Autodesk Fusion 360 part; units mm, degrees
(part 3 of 4)
  spline S780 degree 3 poles (162.707, 0) (162.5525, 0.1099) (162.343, 0.1683) (162.2434, 0.3296) knots 0 0 0 0 1 1 1 1
  spline S781 degree 3 poles (162.2434, 0.3296) (161.8581, 0.9535) (161.6678, 1.6847) (161.2818, 2.3082) knots 0 0 0 0 1 1 1 1
  spline S782 degree 3 poles (161.2818, 2.3082) (160.719, 3.2174) (160.1131, 4.1081) (159.4072, 4.9112) knots 0 0 0 0 1 1 1 1
  spline S783 degree 3 poles (159.4072, 4.9112) (158.7995, 5.6026) (158.0938, 6.2084) (157.3624, 6.7673) knots 0 0 0 0 1 1 1 1
  spline S784 degree 3 poles (157.3624, 6.7673) (156.5565, 7.3833) (155.641, 7.8427) (154.8102, 8.4245) knots 0 0 0 0 1 1 1 1
  spline S785 degree 3 poles (154.8102, 8.4245) (154.6015, 8.5707) (154.3988, 8.7382) (154.2513, 8.9459) knots 0 0 0 0 1 1 1 1
  spline S786 degree 3 poles (154.2513, 8.9459) (154.1313, 9.1149) (154.0733, 9.3238) (154.028, 9.526) knots 0 0 0 0 1 1 1 1
  spline S787 degree 3 poles (154.028, 9.526) (153.9612, 9.8241) (153.9281, 10.1306) (153.9173, 10.4359) knots 0 0 0 0 1 1 1 1
  spline S788 degree 3 poles (153.9173, 10.4359) (153.8511, 12.3143) (153.8373, 14.1943) (153.7972, 16.0734) knots 0 0 0 0 1 1 1 1
  spline S789 degree 3 poles (154.328, 36.0186) (154.1191, 36.017) (153.9103, 36.0154) (153.7014, 36.0138) knots 0 0 0 0 1 1 1 1
  spline S790 degree 3 poles (153.503, 90.7209) (153.3923, 90.7448) (153.2816, 90.7686) (153.1709, 90.7925) knots 0 0 0 0 1 1 1 1
  spline S791 degree 3 poles (153.0996, 107.2371) (153.1846, 106.7302) (153.3367, 106.2301) (153.3546, 105.7164) knots 0 0 0 0 1 1 1 1
  spline S792 degree 3 poles (153.3546, 105.7164) (153.416, 103.9626) (153.3139, 102.2065) (153.337, 100.4517) knots 0 0 0 0 1 1 1 1
  spline S793 degree 3 poles (153.337, 100.4517) (153.369, 98.0177) (153.5698, 95.5852) (153.5198, 93.1515) knots 0 0 0 0 1 1 1 1
  spline S794 degree 3 poles (153.5198, 93.1515) (153.5098, 92.6629) (153.2785, 92.2042) (153.1579, 91.7306) knots 0 0 0 0 1 1 1 1
  spline S795 degree 3 poles (153.0696, 113.8009) (153.1646, 113.374) (153.2945, 112.9533) (153.3547, 112.5201) knots 0 0 0 0 1 1 1 1
  spline S796 degree 3 poles (153.3547, 112.5201) (153.3831, 112.3158) (153.3687, 112.1048) (153.3337, 111.9015) knots 0 0 0 0 1 1 1 1
  spline S797 degree 3 poles (153.3337, 111.9015) (153.2775, 111.5746) (153.1664, 111.2595) (153.0827, 110.9385) knots 0 0 0 0 1 1 1 1
  spline S798 degree 3 poles (152.9654, 140.9767) (153.0459, 140.643) (153.1607, 140.3156) (153.2067, 139.9754) knots 0 0 0 0 1 1 1 1
  spline S799 degree 3 poles (153.2067, 139.9754) (153.2508, 139.6494) (153.2325, 139.3179) (153.2341, 138.9889) knots 0 0 0 0 1 1 1 1
  spline S800 degree 3 poles (153.2341, 138.9889) (153.2588, 133.9022) (153.2897, 128.8155) (153.2858, 123.7287) knots 0 0 0 0 1 1 1 1
  spline S801 degree 3 poles (153.2858, 123.7287) (153.2852, 123.0168) (153.2686, 122.3043) (153.2205, 121.5941) knots 0 0 0 0 1 1 1 1
  spline S802 degree 3 poles (153.2205, 121.5941) (153.1866, 121.0943) (153.0705, 120.6021) (153.04, 120.1021) knots 0 0 0 0 1 1 1 1
  spline S803 degree 3 poles (153.04, 120.1021) (153.0124, 119.6503) (153.0023, 119.1947) (153.0465, 118.7443) knots 0 0 0 0 1 1 1 1
  spline S804 degree 3 poles (153.0465, 118.7443) (153.1022, 118.1763) (153.2777, 117.6248) (153.3386, 117.0573) knots 0 0 0 0 1 1 1 1
  spline S805 degree 3 poles (153.3386, 117.0573) (153.3709, 116.7565) (153.3702, 116.4489) (153.3248, 116.1498) knots 0 0 0 0 1 1 1 1
  spline S806 degree 3 poles (153.3248, 116.1498) (153.2775, 115.8382) (153.1502, 115.544) (153.0629, 115.2411) knots 0 0 0 0 1 1 1 1
  spline S807 degree 3 poles (154.0634, 122.5487) (153.7954, 122.5914) (153.5274, 122.6342) (153.2594, 122.677) knots 0 0 0 0 1 1 1 1
  spline S808 degree 3 poles (152.9512, 147.0062) (153.0349, 146.6532) (153.1573, 146.3072) (153.2024, 145.9472) knots 0 0 0 0 1 1 1 1
  spline S809 degree 3 poles (153.2024, 145.9472) (153.2487, 145.5771) (153.223, 145.2015) (153.2237, 144.8285) knots 0 0 0 0 1 1 1 1
  spline S810 degree 3 poles (153.2237, 144.8285) (153.2242, 144.5201) (153.2505, 144.2085) (153.206, 143.9033) knots 0 0 0 0 1 1 1 1
  spline S811 degree 3 poles (153.206, 143.9033) (153.1619, 143.602) (153.042, 143.3168) (152.96, 143.0235) knots 0 0 0 0 1 1 1 1
  spline S812 degree 3 poles (152.9452, 150.8938) (153.0274, 150.6921) (153.1451, 150.5015) (153.192, 150.2887) knots 0 0 0 0 1 1 1 1
  spline S813 degree 3 poles (153.192, 150.2887) (153.2367, 150.086) (153.2152, 149.874) (153.2156, 149.6664) knots 0 0 0 0 1 1 1 1
  spline S814 degree 3 poles (153.2156, 149.6664) (153.2159, 149.5184) (153.2239, 149.368) (153.1941, 149.223) knots 0 0 0 0 1 1 1 1
  spline S815 degree 3 poles (153.1941, 149.223) (153.1344, 148.9333) (153.0305, 148.6545) (152.9488, 148.3703) knots 0 0 0 0 1 1 1 1
  spline S816 degree 3 poles (156.3329, 165.4136) (156.0015, 165.2513) (155.6952, 165.0222) (155.3388, 164.9267) knots 0 0 0 0 1 1 1 1
  spline S817 degree 3 poles (155.3388, 164.9267) (155.0427, 164.8474) (154.7258, 164.886) (154.4196, 164.9012) knots 0 0 0 0 1 1 1 1
  spline S818 degree 3 poles (154.4196, 164.9012) (154.1292, 164.9157) (153.843, 164.9775) (153.5547, 165.0156) knots 0 0 0 0 1 1 1 1
  spline S819 degree 3 poles (155.7861, 165.1661) (155.9235, 165.0932) (156.044, 164.9681) (156.1982, 164.9473) knots 0 0 0 0 1 1 1 1
  spline S820 degree 3 poles (156.1982, 164.9473) (156.6531, 164.8858) (157.1161, 164.9234) (157.5752, 164.9243) knots 0 0 0 0 1 1 1 1
  spline S821 degree 3 poles (157.5752, 164.9243) (157.8528, 164.9248) (158.1321, 164.9161) (158.4074, 164.9514) knots 0 0 0 0 1 1 1 1
  spline S822 degree 3 poles (158.4074, 164.9514) (158.8796, 165.012) (159.3437, 165.1247) (159.8118, 165.2113) knots 0 0 0 0 1 1 1 1
  spline S823 degree 3 poles (178.3424, 165.3678) (177.9374, 165.3072) (177.5356, 165.2189) (177.1274, 165.1861) knots 0 0 0 0 1 1 1 1
  spline S824 degree 3 poles (177.1274, 165.1861) (176.75, 165.1558) (176.3688, 165.1469) (175.9915, 165.1789) knots 0 0 0 0 1 1 1 1
  spline S825 degree 3 poles (175.9915, 165.1789) (175.5602, 165.2155) (175.1431, 165.3827) (174.7102, 165.391) knots 0 0 0 0 1 1 1 1
  spline S826 degree 3 poles (174.7102, 165.391) (172.3795, 165.4359) (170.0478, 165.2968) (167.717, 165.3382) knots 0 0 0 0 1 1 1 1
  spline S827 degree 3 poles (167.717, 165.3382) (167.2356, 165.3468) (166.767, 165.5072) (166.2867, 165.5408) knots 0 0 0 0 1 1 1 1
  spline S828 degree 3 poles (166.2867, 165.5408) (165.7509, 165.5783) (165.2126, 165.5544) (164.6756, 165.551) knots 0 0 0 0 1 1 1 1
  spline S829 degree 3 poles (164.6756, 165.551) (163.9812, 165.5467) (163.284, 165.5818) (162.5925, 165.5178) knots 0 0 0 0 1 1 1 1
  spline S830 degree 3 poles (162.5925, 165.5178) (162.3658, 165.4968) (162.1614, 165.3716) (161.9459, 165.2984) knots 0 0 0 0 1 1 1 1
  spline S831 degree 3 poles (179.1031, 165.3338) (178.8495, 165.3452) (178.5938, 165.3331) (178.3424, 165.3678) knots 0 0 0 0 1 1 1 1
  spline S832 degree 3 poles (178.3424, 165.3678) (177.8191, 165.44) (177.309, 165.5983) (176.7837, 165.6538) knots 0 0 0 0 1 1 1 1
  spline S833 degree 3 poles (176.7837, 165.6538) (176.47, 165.687) (176.1487, 165.6841) (175.8375, 165.6326) knots 0 0 0 0 1 1 1 1
  spline S834 degree 3 poles (175.8375, 165.6326) (175.6902, 165.6081) (175.5709, 165.498) (175.4375, 165.4307) knots 0 0 0 0 1 1 1 1
  spline S835 degree 3 poles (179.0957, 165.9568) (179.1114, 159.0174) (179.1975, 152.0777) (179.143, 145.1384) knots 0 0 0 0 1 1 1 1
  spline S836 degree 3 poles (179.143, 145.1384) (179.1379, 144.4898) (178.9671, 143.8524) (178.917, 143.2057) knots 0 0 0 0 1 1 1 1
  spline S837 degree 3 poles (178.917, 143.2057) (178.8989, 142.9714) (178.8909, 142.731) (178.9388, 142.5009) knots 0 0 0 0 1 1 1 1
  spline S838 degree 3 poles (178.9388, 142.5009) (179.046, 141.9849) (179.2688, 141.4978) (179.3792, 140.9825) knots 0 0 0 0 1 1 1 1
  spline S839 degree 3 poles (179.3792, 140.9825) (179.43, 140.7456) (179.4179, 140.499) (179.4196, 140.2568) knots 0 0 0 0 1 1 1 1
  spline S840 degree 3 poles (179.4196, 140.2568) (179.4248, 139.496) (179.4847, 138.7306) (179.3998, 137.9747) knots 0 0 0 0 1 1 1 1
  spline S841 degree 3 poles (179.3998, 137.9747) (179.3234, 137.2945) (179.055, 136.6483) (178.9383, 135.974) knots 0 0 0 0 1 1 1 1
  spline S842 degree 3 poles (178.9383, 135.974) (178.8948, 135.7226) (178.9209, 135.4639) (178.9211, 135.2088) knots 0 0 0 0 1 1 1 1
  spline S843 degree 3 poles (178.9211, 135.2088) (178.9271, 127.7745) (178.9353, 120.3402) (178.957, 112.9059) knots 0 0 0 0 1 1 1 1
  spline S844 degree 3 poles (178.957, 112.9059) (178.9581, 112.5277) (178.9443, 112.1473) (178.9892, 111.7717) knots 0 0 0 0 1 1 1 1
  spline S845 degree 3 poles (178.9892, 111.7717) (179.0311, 111.4216) (179.1404, 111.0828) (179.2161, 110.7384) knots 0 0 0 0 1 1 1 1
  spline S846 degree 3 poles (179.143, 145.1384) (179.2272, 144.7257) (179.3417, 144.3182) (179.3955, 143.9005) knots 0 0 0 0 1 1 1 1
  spline S847 degree 3 poles (179.3955, 143.9005) (179.4332, 143.6079) (179.4218, 143.3106) (179.4166, 143.0156) knots 0 0 0 0 1 1 1 1
  spline S848 degree 3 poles (179.4166, 143.0156) (179.4127, 142.797) (179.4165, 142.5747) (179.3684, 142.3615) knots 0 0 0 0 1 1 1 1
  spline S849 degree 3 poles (179.3684, 142.3615) (179.2573, 141.8686) (178.9997, 141.4091) (178.9411, 140.9074) knots 0 0 0 0 1 1 1 1
  spline S850 degree 3 poles (178.9411, 140.9074) (178.8484, 140.1134) (178.9181, 139.3087) (178.9183, 138.5094) knots 0 0 0 0 1 1 1 1
  spline S851 degree 3 poles (178.9183, 138.5094) (178.9184, 138.3273) (178.9065, 138.1423) (178.942, 137.9638) knots 0 0 0 0 1 1 1 1
  spline S852 degree 3 poles (178.942, 137.9638) (179.0571, 137.3857) (179.2568, 136.8265) (179.3685, 136.2478) knots 0 0 0 0 1 1 1 1
  spline S853 degree 3 poles (179.3685, 136.2478) (179.4172, 135.996) (179.4206, 135.7367) (179.4215, 135.4802) knots 0 0 0 0 1 1 1 1
  spline S854 degree 3 poles (179.4215, 135.4802) (179.4469, 128.2535) (179.4502, 121.0268) (179.4474, 113.8001) knots 0 0 0 0 1 1 1 1
  spline S855 degree 3 poles (179.4474, 113.8001) (179.4472, 113.1228) (179.4861, 112.4418) (179.4125, 111.7686) knots 0 0 0 0 1 1 1 1
  spline S856 degree 3 poles (179.4125, 111.7686) (179.3245, 110.9633) (179.0168, 110.1885) (178.9642, 109.3801) knots 0 0 0 0 1 1 1 1
  spline S857 degree 3 poles (178.9642, 109.3801) (178.863, 107.8263) (178.9502, 106.2659) (178.9529, 104.7089) knots 0 0 0 0 1 1 1 1
  spline S858 degree 3 poles (178.9529, 104.7089) (178.9535, 104.3678) (178.9307, 104.0242) (178.9743, 103.686) knots 0 0 0 0 1 1 1 1
  spline S859 degree 3 poles (178.9743, 103.686) (179.0287, 103.2634) (179.1552, 102.8532) (179.2457, 102.4368) knots 0 0 0 0 1 1 1 1
  spline S860 degree 3 poles (179.3943, 127.6548) (179.2509, 127.6546) (179.1075, 127.6543) (178.9641, 127.6541) knots 0 0 0 0 1 1 1 1
  spline S861 degree 3 poles (179.2172, 110.3815) (179.2954, 110.0078) (179.4356, 109.6417) (179.4517, 109.2602) knots 0 0 0 0 1 1 1 1
  spline S862 degree 3 poles (179.4517, 109.2602) (179.5211, 107.6185) (179.5224, 105.9731) (179.4728, 104.3306) knots 0 0 0 0 1 1 1 1
  spline S863 degree 3 poles (179.4728, 104.3306) (179.4536, 103.6951) (179.2605, 103.0724) (179.2457, 102.4368) knots 0 0 0 0 1 1 1 1
  spline S864 degree 3 poles (179.2457, 102.4368) (179.1941, 100.2162) (179.3217, 97.9939) (179.274, 95.7732) knots 0 0 0 0 1 1 1 1
  spline S865 degree 3 poles (179.274, 95.7732) (179.2685, 95.5153) (179.1174, 95.2786) (179.0865, 95.0225) knots 0 0 0 0 1 1 1 1
  spline S866 degree 3 poles (179.0865, 95.0225) (179.0451, 94.6809) (179.059, 94.3346) (179.0585, 93.9905) knots 0 0 0 0 1 1 1 1
  spline S867 degree 3 poles (179.0585, 93.9905) (179.0537, 90.882) (179.0579, 87.7735) (179.0705, 84.665) knots 0 0 0 0 1 1 1 1
  spline S868 degree 3 poles (179.0705, 84.665) (179.0755, 83.4488) (179.0424, 82.2309) (179.1112, 81.0166) knots 0 0 0 0 1 1 1 1
  spline S869 degree 3 poles (179.1112, 81.0166) (179.1447, 80.4248) (179.2882, 79.8443) (179.3767, 79.2582) knots 0 0 0 0 1 1 1 1
  spline S870 degree 3 poles (179.274, 95.7732) (179.3589, 95.4159) (179.5199, 95.0684) (179.5286, 94.7013) knots 0 0 0 0 1 1 1 1
  spline S871 degree 3 poles (179.5286, 94.7013) (179.624, 90.6448) (179.5785, 86.5862) (179.5855, 82.5286) knots 0 0 0 0 1 1 1 1
  spline S872 degree 3 poles (179.5855, 82.5286) (179.5867, 81.862) (179.5956, 81.1942) (179.5532, 80.5289) knots 0 0 0 0 1 1 1 1
  spline S873 degree 3 poles (179.5532, 80.5289) (179.5259, 80.1022) (179.3964, 79.6854) (179.3767, 79.2582) knots 0 0 0 0 1 1 1 1
  spline S874 degree 3 poles (179.3767, 79.2582) (179.3439, 78.5443) (179.4327, 77.8281) (179.3962, 77.1144) knots 0 0 0 0 1 1 1 1
  spline S875 degree 3 poles (179.3962, 77.1144) (179.3745, 76.6904) (179.2124, 76.2799) (179.2027, 75.8554) knots 0 0 0 0 1 1 1 1
  spline S876 degree 3 poles (179.2027, 75.8554) (179.1504, 73.5649) (179.1994, 71.2732) (179.2105, 68.9821) knots 0 0 0 0 1 1 1 1
  spline S877 degree 3 poles (179.2105, 68.9821) (179.2136, 68.3531) (179.1876, 67.7218) (179.2452, 67.0955) knots 0 0 0 0 1 1 1 1
  spline S878 degree 3 poles (179.2452, 67.0955) (179.2874, 66.6365) (179.4209, 66.1907) (179.5088, 65.7383) knots 0 0 0 0 1 1 1 1
  spline S879 degree 3 poles (179.437, 69.1097) (179.528, 68.7981) (179.6191, 68.4865) (179.7101, 68.1749) knots 0 0 0 0 1 1 1 1
  spline S880 degree 3 poles (179.5184, 64.722) (179.4564, 64.4417) (179.3646, 64.1664) (179.3325, 63.8811) knots 0 0 0 0 1 1 1 1
  spline S881 degree 3 poles (179.3325, 63.8811) (179.2722, 63.3457) (179.1737, 62.8017) (179.242, 62.2673) knots 0 0 0 0 1 1 1 1
  spline S882 degree 3 poles (179.242, 62.2673) (179.3331, 61.5535) (179.6394, 60.8835) (179.8049, 60.1831) knots 0 0 0 0 1 1 1 1
  spline S883 degree 3 poles (179.8049, 60.1831) (179.833, 60.0641) (179.8201, 59.9389) (179.8211, 59.8165) knots 0 0 0 0 1 1 1 1
  spline S884 degree 3 poles (179.8211, 59.8165) (179.844, 57.0288) (179.867, 54.241) (179.8765, 51.4531) knots 0 0 0 0 1 1 1 1
  spline S885 degree 3 poles (179.8765, 51.4531) (179.8774, 51.2037) (179.8863, 50.9523) (179.8523, 50.7052) knots 0 0 0 0 1 1 1 1
  spline S886 degree 3 poles (179.8523, 50.7052) (179.81, 50.397) (179.6854, 50.1033) (179.6485, 49.7944) knots 0 0 0 0 1 1 1 1
  spline S887 degree 3 poles (179.6485, 49.7944) (179.6191, 49.5484) (179.6525, 49.2989) (179.6548, 49.0512) knots 0 0 0 0 1 1 1 1
  spline S888 degree 3 poles (179.6548, 49.0512) (179.657, 48.8038) (179.6345, 48.555) (179.6618, 48.3091) knots 0 0 0 0 1 1 1 1
  spline S889 degree 3 poles (179.6618, 48.3091) (179.7288, 47.7071) (179.9183, 47.1183) (179.9372, 46.5128) knots 0 0 0 0 1 1 1 1
  spline S890 degree 3 poles (179.9372, 46.5128) (180.0188, 43.89) (180.0047, 41.2644) (179.9627, 38.6406) knots 0 0 0 0 1 1 1 1
  spline S891 degree 3 poles (179.9627, 38.6406) (179.9546, 38.1306) (179.7698, 37.6304) (179.7869, 37.1206) knots 0 0 0 0 1 1 1 1
  spline S892 degree 3 poles (179.7869, 37.1206) (179.7941, 36.9044) (179.9871, 36.7317) (180.0336, 36.5204) knots 0 0 0 0 1 1 1 1
  spline S893 degree 3 poles (180.0336, 36.5204) (180.083, 36.2966) (180.0682, 36.063) (180.0704, 35.8337) knots 0 0 0 0 1 1 1 1
  spline S894 degree 3 poles (180.0704, 35.8337) (180.0975, 32.9366) (180.1603, 30.0391) (180.1215, 27.1421) knots 0 0 0 0 1 1 1 1
  spline S895 degree 3 poles (180.1215, 27.1421) (180.1103, 26.304) (179.961, 25.4728) (179.9205, 24.6356) knots 0 0 0 0 1 1 1 1
  spline S896 degree 3 poles (179.9205, 24.6356) (179.8989, 24.1883) (179.9658, 23.7391) (179.9354, 23.2923) knots 0 0 0 0 1 1 1 1
  spline S897 degree 3 poles (179.9354, 23.2923) (179.8975, 22.7363) (179.7263, 22.192) (179.7161, 21.6348) knots 0 0 0 0 1 1 1 1
  spline S898 degree 3 poles (179.7161, 21.6348) (179.6659, 18.9022) (179.7839, 16.1686) (179.7544, 13.4356) knots 0 0 0 0 1 1 1 1
  spline S899 degree 3 poles (179.7544, 13.4356) (179.7404, 12.1407) (179.7624, 10.8372) (179.5858, 9.5542) knots 0 0 0 0 1 1 1 1
  spline S900 degree 3 poles (179.5858, 9.5542) (179.533, 9.1713) (179.2463, 8.8596) (179.0766, 8.5122) knots 0 0 0 0 1 1 1 1
  spline S901 degree 3 poles (179.8049, 60.1831) (179.7736, 60.8021) (179.7119, 61.4203) (179.7109, 62.04) knots 0 0 0 0 1 1 1 1
  spline S902 degree 3 poles (179.7109, 62.04) (179.71, 62.6052) (179.8399, 63.1694) (179.7994, 63.7331) knots 0 0 0 0 1 1 1 1
  spline S903 degree 3 poles (179.7994, 63.7331) (179.7749, 64.0749) (179.5675, 64.3829) (179.5184, 64.722) knots 0 0 0 0 1 1 1 1
  spline S904 degree 3 poles (179.5184, 64.722) (179.4698, 65.0573) (179.4807, 65.4007) (179.5088, 65.7383) knots 0 0 0 0 1 1 1 1
  spline S905 degree 3 poles (179.5088, 65.7383) (179.552, 66.2562) (179.7233, 66.7618) (179.7316, 67.2815) knots 0 0 0 0 1 1 1 1
  spline S906 degree 3 poles (179.7316, 67.2815) (179.7767, 70.0737) (179.6986, 72.8666) (179.669, 75.6591) knots 0 0 0 0 1 1 1 1
  spline S907 degree 3 poles (179.669, 75.6591) (179.667, 75.8432) (179.6709, 76.0295) (179.637, 76.2104) knots 0 0 0 0 1 1 1 1
  spline S908 degree 3 poles (179.637, 76.2104) (179.5795, 76.5169) (179.4764, 76.8131) (179.3962, 77.1144) knots 0 0 0 0 1 1 1 1
  spline S909 degree 3 poles (179.7109, 62.04) (179.5863, 61.3671) (179.4333, 60.6988) (179.3371, 60.0213) knots 0 0 0 0 1 1 1 1
  spline S910 degree 3 poles (179.3371, 60.0213) (179.3041, 59.7891) (179.3236, 59.5523) (179.3242, 59.3178) knots 0 0 0 0 1 1 1 1
  spline S911 degree 3 poles (179.3242, 59.3178) (179.3315, 56.6374) (179.3422, 53.9569) (179.3608, 51.2766) knots 0 0 0 0 1 1 1 1
  spline S912 degree 3 poles (179.3608, 51.2766) (179.3622, 51.0735) (179.3456, 50.8671) (179.3843, 50.6678) knots 0 0 0 0 1 1 1 1
  spline S913 degree 3 poles (179.3843, 50.6678) (179.4423, 50.3692) (179.5605, 50.0855) (179.6485, 49.7944) knots 0 0 0 0 1 1 1 1
  spline S914 degree 3 poles (179.5684, 52.0486) (179.6531, 52.577) (179.7378, 53.1054) (179.8225, 53.6339) knots 0 0 0 0 1 1 1 1
  spline S915 degree 3 poles (179.6618, 48.3091) (179.5981, 47.8001) (179.4823, 47.2948) (179.4706, 46.7819) knots 0 0 0 0 1 1 1 1
  spline S916 degree 3 poles (179.4706, 46.7819) (179.4249, 44.7749) (179.4795, 42.7669) (179.4898, 40.7594) knots 0 0 0 0 1 1 1 1
  spline S917 degree 3 poles (179.4898, 40.7594) (179.4921, 40.3029) (179.4713, 39.8449) (179.5084, 39.3899) knots 0 0 0 0 1 1 1 1
  spline S918 degree 3 poles (179.5084, 39.3899) (179.5705, 38.6303) (179.6941, 37.877) (179.7869, 37.1206) knots 0 0 0 0 1 1 1 1
  spline S919 degree 3 poles (179.7332, 39.2245) (179.7511, 38.5232) (179.8199, 37.8214) (179.7869, 37.1206) knots 0 0 0 0 1 1 1 1
  spline S920 degree 3 poles (179.7869, 37.1206) (179.7752, 36.8734) (179.6363, 36.6468) (179.6003, 36.4019) knots 0 0 0 0 1 1 1 1
  spline S921 degree 3 poles (179.6003, 36.4019) (179.5668, 36.1741) (179.5794, 35.9418) (179.5798, 35.7116) knots 0 0 0 0 1 1 1 1
  spline S922 degree 3 poles (179.5798, 35.7116) (179.584, 33.0281) (179.5963, 30.3446) (179.6142, 27.6612) knots 0 0 0 0 1 1 1 1
  spline S923 degree 3 poles (179.6142, 27.6612) (179.6171, 27.2251) (179.5982, 26.787) (179.6421, 26.3531) knots 0 0 0 0 1 1 1 1
  spline S924 degree 3 poles (179.6421, 26.3531) (179.7006, 25.7761) (179.8277, 25.2081) (179.9205, 24.6356) knots 0 0 0 0 1 1 1 1
  spline S925 degree 3 poles (179.159, 20.8424) (179.3482, 20.7545) (179.5373, 20.6666) (179.7264, 20.5787) knots 0 0 0 0 1 1 1 1
  spline S926 degree 3 poles (179.9354, 23.2923) (180.0299, 22.7609) (180.2008, 22.2375) (180.2189, 21.698) knots 0 0 0 0 1 1 1 1
  spline S927 degree 3 poles (180.2189, 21.698) (180.3105, 18.9754) (180.2195, 16.2496) (180.2638, 13.5259) knots 0 0 0 0 1 1 1 1
  spline S928 degree 3 poles (180.2638, 13.5259) (180.2764, 12.7552) (180.3714, 11.9875) (180.3893, 11.2169) knots 0 0 0 0 1 1 1 1
  spline S929 degree 3 poles (180.3893, 11.2169) (180.3955, 10.9526) (180.3817, 10.6859) (180.3359, 10.4256) knots 0 0 0 0 1 1 1 1
  spline S930 degree 3 poles (180.3359, 10.4256) (180.2773, 10.0927) (180.2827, 9.7136) (180.0775, 9.445) knots 0 0 0 0 1 1 1 1
  spline S931 degree 3 poles (180.0775, 9.445) (179.6468, 8.8809) (179.0701, 8.437) (178.4973, 8.0181) knots 0 0 0 0 1 1 1 1
  spline S932 degree 3 poles (178.4973, 8.0181) (178.0078, 7.6601) (177.3899, 7.4999) (176.9104, 7.1287) knots 0 0 0 0 1 1 1 1
  spline S933 degree 3 poles (176.9104, 7.1287) (176.1096, 6.5088) (175.3972, 5.7809) (174.6817, 5.0643) knots 0 0 0 0 1 1 1 1
  spline S934 degree 3 poles (174.6817, 5.0643) (174.3169, 4.6989) (173.9616, 4.3167) (173.6744, 3.8876) knots 0 0 0 0 1 1 1 1
  spline S935 degree 3 poles (173.6744, 3.8876) (172.847, 2.6516) (172.1222, 1.35) (171.3461, 0.0812) knots 0 0 0 0 1 1 1 1
  spline S936 degree 3 poles (155.3539, 33.3788) (155.3058, 33.3487) (155.2401, 33.3364) (155.2094, 33.2885) knots 0 0 0 0 1 1 1 1
  spline S937 degree 3 poles (155.2094, 33.2885) (155.1747, 33.2342) (155.186, 33.1617) (155.1743, 33.0982) knots 0 0 0 0 1 1 1 1
  spline S938 degree 3 poles (167.9554, 45.7488) (167.8434, 46.0195) (167.7314, 46.2902) (167.6194, 46.5608) knots 0 0 0 0 1 1 1 1
  spline S939 degree 3 poles (168.3945, 150.5926) (168.4008, 150.5154) (168.407, 150.4381) (168.4133, 150.3608) knots 0 0 0 0 1 1 1 1
  spline S940 degree 3 poles (175.1064, 61.9868) (175.0738, 61.7404) (175.1218, 61.4689) (175.0086, 61.2477) knots 0 0 0 0 1 1 1 1
  spline S941 degree 3 poles (175.0086, 61.2477) (174.8804, 60.9973) (174.5698, 60.8813) (174.4191, 60.6438) knots 0 0 0 0 1 1 1 1
  spline S942 degree 3 poles (174.4191, 60.6438) (174.3245, 60.4947) (174.3385, 60.3) (174.2982, 60.1281) knots 0 0 0 0 1 1 1 1
  spline S943 degree 3 poles (201.6005, 14.2898) (201.7429, 14.4728) (201.8853, 14.6559) (202.0277, 14.8389) knots 0 0 0 0 1 1 1 1
  spline S944 degree 3 poles (201.7004, 11.2556) (201.7672, 12.1989) (201.7949, 13.1459) (201.901, 14.0857) knots 0 0 0 0 1 1 1 1
  spline S945 degree 3 poles (201.901, 14.0857) (201.9634, 14.6386) (202.1324, 15.1754) (202.205, 15.7271) knots 0 0 0 0 1 1 1 1
  spline S946 degree 3 poles (202.205, 15.7271) (202.2883, 16.3607) (202.2848, 17.0038) (202.3682, 17.6375) knots 0 0 0 0 1 1 1 1
  spline S947 degree 3 poles (202.3682, 17.6375) (202.5492, 19.012) (202.8189, 20.374) (202.9978, 21.7488) knots 0 0 0 0 1 1 1 1
  spline S948 degree 3 poles (202.9978, 21.7488) (203.1159, 22.6558) (203.2016, 23.5675) (203.2591, 24.4803) knots 0 0 0 0 1 1 1 1
  spline S949 degree 3 poles (203.2591, 24.4803) (203.2822, 24.8477) (203.2461, 25.2165) (203.2395, 25.5846) knots 0 0 0 0 1 1 1 1
  spline S950 degree 3 poles (202.7573, 15.0316) (202.5472, 15.0387) (202.337, 15.0458) (202.1269, 15.0529) knots 0 0 0 0 1 1 1 1
  spline S951 degree 3 poles (203.5642, 54.0188) (203.5939, 53.7748) (203.6827, 53.5309) (203.6533, 53.2868) knots 0 0 0 0 1 1 1 1
  spline S952 degree 3 poles (203.6533, 53.2868) (203.6053, 52.8871) (203.3836, 52.5212) (203.3362, 52.1215) knots 0 0 0 0 1 1 1 1
  spline S953 degree 3 poles (203.3362, 52.1215) (203.252, 51.4117) (203.3296, 50.6899) (203.2611, 49.9785) knots 0 0 0 0 1 1 1 1
  spline S954 degree 3 poles (203.2611, 49.9785) (203.2306, 49.662) (203.1138, 49.3599) (203.0401, 49.0506) knots 0 0 0 0 1 1 1 1
  spline S955 degree 3 poles (203.1464, 78.6257) (203.0244, 78.6678) (202.8265, 78.6314) (202.7804, 78.7519) knots 0 0 0 0 1 1 1 1
  spline S956 degree 3 poles (202.7804, 78.7519) (202.5119, 79.4526) (202.4328, 80.2118) (202.259, 80.9418) knots 0 0 0 0 1 1 1 1
  spline S957 degree 3 poles (203.0903, 79.9439) (202.8623, 80.0109) (202.6342, 80.078) (202.4061, 80.1451) knots 0 0 0 0 1 1 1 1
  spline S958 degree 3 poles (203.4352, 136.8282) (203.3092, 136.8405) (203.1833, 136.8529) (203.0573, 136.8652) knots 0 0 0 0 1 1 1 1
  spline S959 degree 3 poles (203.5465, 137.3313) (203.3816, 137.3599) (203.2167, 137.3885) (203.0519, 137.4172) knots 0 0 0 0 1 1 1 1
  spline S960 degree 3 poles (203.0116, 127.0535) (203.1109, 127.0971) (203.226, 127.1152) (203.3096, 127.1843) knots 0 0 0 0 1 1 1 1
  spline S961 degree 3 poles (203.3096, 127.1843) (203.3547, 127.2217) (203.3952, 127.297) (203.3695, 127.3497) knots 0 0 0 0 1 1 1 1
  spline S962 degree 3 poles (203.3695, 127.3497) (203.2464, 127.6017) (202.9687, 127.7723) (202.8908, 128.0417) knots 0 0 0 0 1 1 1 1
  spline S963 degree 3 poles (202.8908, 128.0417) (202.708, 128.6747) (202.631, 129.3391) (202.6047, 129.9974) knots 0 0 0 0 1 1 1 1
  spline S964 degree 3 poles (202.6047, 129.9974) (202.5783, 130.6583) (202.6457, 131.322) (202.7337, 131.9776) knots 0 0 0 0 1 1 1 1
  spline S965 degree 3 poles (202.7337, 131.9776) (202.793, 132.4192) (202.9817, 132.8366) (203.0451, 133.2776) knots 0 0 0 0 1 1 1 1
  spline S966 degree 3 poles (203.0451, 133.2776) (203.0944, 133.6198) (203.1305, 133.974) (203.0701, 134.3144) knots 0 0 0 0 1 1 1 1
  spline S967 degree 3 poles (203.0701, 134.3144) (202.9555, 134.9608) (202.622, 135.5578) (202.5258, 136.2072) knots 0 0 0 0 1 1 1 1
  spline S968 degree 3 poles (202.5258, 136.2072) (202.4425, 136.7691) (202.5061, 137.3441) (202.5373, 137.9113) knots 0 0 0 0 1 1 1 1
  spline S969 degree 3 poles (202.5373, 137.9113) (202.5447, 138.0455) (202.5422, 138.2098) (202.6409, 138.3011) knots 0 0 0 0 1 1 1 1
  spline S970 degree 3 poles (202.6409, 138.3011) (202.8738, 138.5165) (203.1589, 138.7005) (203.468, 138.7718) knots 0 0 0 0 1 1 1 1
  spline S971 degree 3 poles (203.468, 138.7718) (204.0811, 138.9132) (204.7202, 138.9322) (205.3493, 138.9257) knots 0 0 0 0 1 1 1 1
  spline S972 degree 3 poles (205.3493, 138.9257) (205.9941, 138.9192) (206.6294, 138.7426) (207.2742, 138.733) knots 0 0 0 0 1 1 1 1
  spline S973 degree 3 poles (207.2742, 138.733) (208.4626, 138.7154) (209.6549, 138.7319) (210.8381, 138.8443) knots 0 0 0 0 1 1 1 1
  spline S974 degree 3 poles (210.8381, 138.8443) (211.1451, 138.8734) (211.6578, 139.4581) (211.7096, 139.1542) knots 0 0 0 0 1 1 1 1
  spline S975 degree 3 poles (211.7096, 139.1542) (211.9878, 137.5202) (211.6116, 135.8396) (211.6319, 134.1822) knots 0 0 0 0 1 1 1 1
  spline S976 degree 3 poles (211.6319, 134.1822) (211.6358, 133.8683) (211.679, 133.5489) (211.782, 133.2523) knots 0 0 0 0 1 1 1 1
  spline S977 degree 3 poles (211.782, 133.2523) (211.9609, 132.7369) (212.2409, 132.2623) (212.4704, 131.7674) knots 0 0 0 0 1 1 1 1
  spline S978 degree 3 poles (212.9028, 92.7168) (212.9037, 94.5151) (212.9538, 96.3141) (212.9056, 98.1117) knots 0 0 0 0 1 1 1 1
  spline S979 degree 3 poles (212.9056, 98.1117) (212.9004, 98.3051) (212.8368, 98.4995) (212.7431, 98.6688) knots 0 0 0 0 1 1 1 1
  spline S980 degree 3 poles (212.7431, 98.6688) (212.5787, 98.9661) (212.2822, 99.1826) (212.1421, 99.4921) knots 0 0 0 0 1 1 1 1
  spline S981 degree 3 poles (212.1421, 99.4921) (212.0578, 99.6783) (212.0949, 99.8989) (212.0938, 100.1033) knots 0 0 0 0 1 1 1 1
  spline S982 degree 3 poles (212.0938, 100.1033) (212.0381, 110.5035) (211.944, 120.9038) (211.9717, 131.304) knots 0 0 0 0 1 1 1 1
  spline S983 degree 3 poles (211.9717, 131.304) (211.9737, 132.0728) (212.1126, 132.8351) (212.183, 133.6005) knots 0 0 0 0 1 1 1 1
  spline S984 degree 3 poles (212.4599, 130.4526) (212.3136, 130.4441) (212.1673, 130.4356) (212.021, 130.4271) knots 0 0 0 0 1 1 1 1
  spline S985 degree 3 poles (212.1028, 102.892) (211.8395, 103.2671) (211.5048, 103.6012) (211.3131, 104.0174) knots 0 0 0 0 1 1 1 1
  spline S986 degree 3 poles (211.3131, 104.0174) (211.2701, 104.1106) (211.362, 104.2564) (211.4595, 104.2884) knots 0 0 0 0 1 1 1 1
  spline S987 degree 3 poles (211.4595, 104.2884) (211.6536, 104.352) (211.9462, 104.4272) (212.072, 104.2662) knots 0 0 0 0 1 1 1 1
  spline S988 degree 3 poles (212.072, 104.2662) (212.2335, 104.0595) (212.2581, 103.6822) (212.0917, 103.4792) knots 0 0 0 0 1 1 1 1
  spline S989 degree 3 poles (212.0917, 103.4792) (211.905, 103.2515) (211.523, 103.3263) (211.2386, 103.2499) knots 0 0 0 0 1 1 1 1
  spline S990 degree 3 poles (210.7639, 140.0672) (210.9094, 140.0406) (211.1137, 140.1073) (211.2004, 139.9875) knots 0 0 0 0 1 1 1 1
  spline S991 degree 3 poles (211.2004, 139.9875) (211.5901, 139.4488) (212.0056, 138.8678) (212.1067, 138.2106) knots 0 0 0 0 1 1 1 1
  spline S992 degree 3 poles (212.1067, 138.2106) (212.3404, 136.6916) (212.0943, 135.1349) (212.183, 133.6005) knots 0 0 0 0 1 1 1 1
  spline S993 degree 3 poles (212.183, 133.6005) (212.2213, 132.9373) (212.4727, 132.2949) (212.4869, 131.6307) knots 0 0 0 0 1 1 1 1
  spline S994 degree 3 poles (212.4869, 131.6307) (212.5822, 127.1495) (212.4738, 122.6661) (212.5111, 118.184) knots 0 0 0 0 1 1 1 1
  spline S995 degree 3 poles (212.5111, 118.184) (212.5608, 112.2137) (212.7072, 106.2444) (212.7481, 100.274) knots 0 0 0 0 1 1 1 1
  spline S996 degree 3 poles (212.7481, 100.274) (212.7515, 99.7761) (212.6788, 99.2806) (212.6441, 98.7839) knots 0 0 0 0 1 1 1 1
  spline S997 degree 3 poles (208.6453, 139.1047) (208.7903, 139.1753) (208.92, 139.2992) (209.0804, 139.3164) knots 0 0 0 0 1 1 1 1
  spline S998 degree 3 poles (209.0804, 139.3164) (209.9085, 139.4054) (210.7448, 139.3852) (211.5769, 139.4196) knots 0 0 0 0 1 1 1 1
  spline S999 degree 3 poles (209.078, 138.8387) (208.582, 138.9675) (208.0971, 139.1515) (207.5899, 139.2252) knots 0 0 0 0 1 1 1 1
  spline S1000 degree 3 poles (207.5899, 139.2252) (207.2733, 139.2712) (206.9452, 139.2529) (206.6307, 139.1944) knots 0 0 0 0 1 1 1 1
  spline S1001 degree 3 poles (206.6307, 139.1944) (206.4806, 139.1665) (206.3796, 139.0037) (206.2302, 138.9724) knots 0 0 0 0 1 1 1 1
  spline S1002 degree 3 poles (206.2302, 138.9724) (205.9424, 138.9121) (205.6429, 138.9413) (205.3493, 138.9257) knots 0 0 0 0 1 1 1 1
  spline S1003 degree 3 poles (203.468, 138.7718) (203.3157, 138.5294) (203.0604, 138.3266) (203.011, 138.0445) knots 0 0 0 0 1 1 1 1
  spline S1004 degree 3 poles (203.011, 138.0445) (202.9046, 137.4373) (203.0864, 136.8076) (203.0166, 136.1951) knots 0 0 0 0 1 1 1 1
  spline S1005 degree 3 poles (203.0166, 136.1951) (202.943, 135.548) (202.6915, 134.9321) (202.5834, 134.2899) knots 0 0 0 0 1 1 1 1
  spline S1006 degree 3 poles (202.5834, 134.2899) (202.5111, 133.8605) (202.5425, 133.4184) (202.4768, 132.988) knots 0 0 0 0 1 1 1 1
  spline S1007 degree 3 poles (202.4768, 132.988) (202.3924, 132.4352) (202.1575, 131.9045) (202.1341, 131.3458) knots 0 0 0 0 1 1 1 1
  spline S1008 degree 3 poles (202.1341, 131.3458) (201.9841, 127.7593) (201.9686, 124.168) (201.9578, 120.5784) knots 0 0 0 0 1 1 1 1
  spline S1009 degree 3 poles (201.9578, 120.5784) (201.9403, 114.7551) (202.0558, 108.932) (202.0493, 103.1087) knots 0 0 0 0 1 1 1 1
  spline S1010 degree 3 poles (202.0493, 103.1087) (202.0491, 102.8475) (201.9357, 102.5943) (201.9376, 102.3331) knots 0 0 0 0 1 1 1 1
  spline S1011 degree 3 poles (201.9376, 102.3331) (201.9407, 101.9374) (202.0589, 101.5483) (202.0642, 101.1526) knots 0 0 0 0 1 1 1 1
  spline S1012 degree 3 poles (202.0642, 101.1526) (202.0785, 100.0886) (201.9886, 99.0251) (201.9961, 97.961) knots 0 0 0 0 1 1 1 1
  spline S1013 degree 3 poles (201.9961, 97.961) (202.0072, 96.4124) (202.0297, 94.8628) (202.1201, 93.3168) knots 0 0 0 0 1 1 1 1
  spline S1014 degree 3 poles (202.1201, 93.3168) (202.1268, 93.2022) (202.2586, 93.1263) (202.2854, 93.0146) knots 0 0 0 0 1 1 1 1
  spline S1015 degree 3 poles (202.2854, 93.0146) (202.3328, 92.8164) (202.3777, 92.6053) (202.338, 92.4054) knots 0 0 0 0 1 1 1 1
  spline S1016 degree 3 poles (202.338, 92.4054) (202.3096, 92.2625) (202.0963, 92.1894) (202.0924, 92.0437) knots 0 0 0 0 1 1 1 1
  spline S1017 degree 3 poles (202.0924, 92.0437) (202.0348, 89.9151) (202.1084, 87.7847) (202.1553, 85.6558) knots 0 0 0 0 1 1 1 1
  spline S1018 degree 3 poles (202.1553, 85.6558) (202.3375, 77.397) (202.6307, 69.1407) (202.7795, 60.8812) knots 0 0 0 0 1 1 1 1
  spline S1019 degree 3 poles (202.7795, 60.8812) (202.8007, 59.7041) (202.6693, 58.5284) (202.6653, 57.351) knots 0 0 0 0 1 1 1 1
  spline S1020 degree 3 poles (202.6653, 57.351) (202.6581, 55.2288) (202.6536, 53.105) (202.7459, 50.9847) knots 0 0 0 0 1 1 1 1
  spline S1021 degree 3 poles (202.7459, 50.9847) (202.7809, 50.1814) (203.0383, 49.3953) (203.0469, 48.5913) knots 0 0 0 0 1 1 1 1
  spline S1022 degree 3 poles (203.0469, 48.5913) (203.0564, 47.7144) (203.004, 46.8249) (202.7999, 45.972) knots 0 0 0 0 1 1 1 1
  spline S1023 degree 3 poles (202.7999, 45.972) (202.7571, 45.7934) (202.4689, 45.7964) (202.3454, 45.6605) knots 0 0 0 0 1 1 1 1
  spline S1024 degree 3 poles (202.3454, 45.6605) (202.3111, 45.6227) (202.3447, 45.5472) (202.3813, 45.5117) knots 0 0 0 0 1 1 1 1
  spline S1025 degree 3 poles (202.3813, 45.5117) (202.5096, 45.3872) (202.7713, 45.3737) (202.8187, 45.2013) knots 0 0 0 0 1 1 1 1
  spline S1026 degree 3 poles (202.8187, 45.2013) (202.9862, 44.5914) (202.9503, 43.9426) (202.9857, 43.3111) knots 0 0 0 0 1 1 1 1
  spline S1027 degree 3 poles (202.9857, 43.3111) (203.0527, 42.1176) (203.103, 40.9229) (203.1259, 39.7278) knots 0 0 0 0 1 1 1 1
  spline S1028 degree 3 poles (203.1259, 39.7278) (203.2107, 35.3119) (203.2735, 30.8955) (203.309, 26.4789) knots 0 0 0 0 1 1 1 1
  spline S1029 degree 3 poles (203.309, 26.4789) (203.3114, 26.1799) (203.3216, 25.8721) (203.2395, 25.5846) knots 0 0 0 0 1 1 1 1
  spline S1030 degree 3 poles (203.2395, 25.5846) (203.1417, 25.2419) (202.8464, 24.9699) (202.7785, 24.62) knots 0 0 0 0 1 1 1 1
  spline S1031 degree 3 poles (202.7785, 24.62) (202.433, 22.8391) (202.3236, 21.0189) (202.0074, 19.2326) knots 0 0 0 0 1 1 1 1
  spline S1032 degree 3 poles (202.0074, 19.2326) (201.4173, 15.8986) (200.716, 12.5851) (200.0603, 9.2634) knots 0 0 0 0 1 1 1 1
  spline S1033 degree 3 poles (200.0603, 9.2634) (200.0396, 9.1583) (200.0281, 9.0475) (199.9784, 8.9527) knots 0 0 0 0 1 1 1 1
  spline S1034 degree 3 poles (199.9784, 8.9527) (199.8424, 8.6935) (199.6294, 8.4775) (199.5083, 8.211) knots 0 0 0 0 1 1 1 1
  spline S1035 degree 3 poles (199.5083, 8.211) (199.2882, 7.7272) (199.0103, 7.2428) (198.96, 6.7137) knots 0 0 0 0 1 1 1 1
  spline S1036 degree 3 poles (198.96, 6.7137) (198.8522, 5.5813) (198.9747, 4.4377) (199.041, 3.3021) knots 0 0 0 0 1 1 1 1
  spline S1037 degree 3 poles (199.041, 3.3021) (199.0745, 2.7291) (198.7987, 1.937) (199.259, 1.5942) knots 0 0 0 0 1 1 1 1
  spline S1038 degree 3 poles (199.259, 1.5942) (199.592, 1.3463) (199.7593, 2.2714) (199.9012, 2.6616) knots 0 0 0 0 1 1 1 1
  spline S1039 degree 3 poles (199.9012, 2.6616) (200.017, 2.9799) (200.0057, 3.3329) (200.0144, 3.6715) knots 0 0 0 0 1 1 1 1
  spline S1040 degree 3 poles (200.0144, 3.6715) (200.0421, 4.7538) (200.1303, 5.8435) (200.0103, 6.9196) knots 0 0 0 0 1 1 1 1
  spline S1041 degree 3 poles (200.0103, 6.9196) (199.9591, 7.3786) (199.6676, 8.6446) (199.5083, 8.211) knots 0 0 0 0 1 1 1 1
  spline S1042 degree 3 poles (199.5083, 8.211) (199.1749, 7.304) (199.4191, 6.2797) (199.42, 5.3133) knots 0 0 0 0 1 1 1 1
  spline S1043 degree 3 poles (199.42, 5.3133) (199.4206, 4.6459) (199.5723, 3.978) (199.5128, 3.3132) knots 0 0 0 0 1 1 1 1
  spline S1044 degree 3 poles (199.5128, 3.3132) (199.4279, 2.3645) (199.2289, 1.4259) (198.9897, 0.5038) knots 0 0 0 0 1 1 1 1
  spline S1045 degree 3 poles (198.9897, 0.5038) (198.9603, 0.3905) (198.8129, 0.3503) (198.7245, 0.2736) knots 0 0 0 0 1 1 1 1
  spline S1046 degree 3 poles (200.7263, 104.614) (201.1428, 104.455) (201.5593, 104.2959) (201.9757, 104.1369) knots 0 0 0 0 1 1 1 1
  spline S1047 degree 3 poles (201.3153, 102.4303) (201.5259, 102.4686) (201.7365, 102.5069) (201.9471, 102.5452) knots 0 0 0 0 1 1 1 1
  spline S1048 degree 3 poles (201.2553, 99.9044) (201.4633, 99.8153) (201.7476, 99.8212) (201.8791, 99.6371) knots 0 0 0 0 1 1 1 1
  spline S1049 degree 3 poles (201.8791, 99.6371) (202.0426, 99.4085) (201.9852, 99.0851) (202.0383, 98.8091) knots 0 0 0 0 1 1 1 1
  spline S1050 degree 3 poles (201.1676, 99.0179) (201.4509, 98.9913) (201.7342, 98.9648) (202.0175, 98.9382) knots 0 0 0 0 1 1 1 1
  spline S1051 degree 3 poles (201.3848, 97.8007) (201.5863, 97.8244) (201.7878, 97.8482) (201.9893, 97.8719) knots 0 0 0 0 1 1 1 1
  spline S1052 degree 3 poles (201.2818, 86.5083) (201.5709, 86.4047) (201.8601, 86.3011) (202.1492, 86.1975) knots 0 0 0 0 1 1 1 1
  spline S1053 degree 3 poles (201.1347, 60.9857) (201.2073, 61.0205) (201.273, 61.0778) (201.3526, 61.0902) knots 0 0 0 0 1 1 1 1
  spline S1054 degree 3 poles (201.3526, 61.0902) (201.8135, 61.1621) (202.2804, 61.1879) (202.7444, 61.2368) knots 0 0 0 0 1 1 1 1
  spline S1055 degree 3 poles (203.8551, 26.0857) (203.8302, 29.7763) (203.852, 33.4675) (203.7804, 37.1575) knots 0 0 0 0 1 1 1 1
  spline S1056 degree 3 poles (203.7804, 37.1575) (203.7425, 39.1095) (203.6331, 41.0596) (203.5265, 43.0091) knots 0 0 0 0 1 1 1 1
  spline S1057 degree 3 poles (203.5265, 43.0091) (203.5041, 43.4172) (203.4117, 43.8197) (203.3935, 44.228) knots 0 0 0 0 1 1 1 1
  spline S1058 degree 3 poles (203.3935, 44.228) (203.3534, 45.1241) (203.4225, 46.0245) (203.3515, 46.9186) knots 0 0 0 0 1 1 1 1
  spline S1059 degree 3 poles (203.3515, 46.9186) (203.3066, 47.4836) (203.1484, 48.0338) (203.0469, 48.5913) knots 0 0 0 0 1 1 1 1
  spline S1060 degree 3 poles (211.6011, 16.851) (211.4478, 16.9051) (211.2801, 16.9288) (211.1413, 17.0133) knots 0 0 0 0 1 1 1 1
  spline S1061 degree 3 poles (211.1413, 17.0133) (211.0459, 17.0714) (210.9943, 17.1813) (210.9208, 17.2654) knots 0 0 0 0 1 1 1 1
  spline S1062 degree 3 poles (218.3881, 2.1498) (218.2337, 2.4399) (218.0792, 2.7299) (217.9248, 3.02) knots 0 0 0 0 1 1 1 1
  spline S1063 degree 3 poles (217.1116, 9.4815) (217.2983, 9.0619) (217.5072, 8.6515) (217.6719, 8.2228) knots 0 0 0 0 1 1 1 1
  spline S1064 degree 3 poles (217.6719, 8.2228) (217.7381, 8.0502) (217.7753, 7.8665) (217.8019, 7.6836) knots 0 0 0 0 1 1 1 1
  spline S1065 degree 3 poles (217.8019, 7.6836) (217.8948, 7.0467) (217.9956, 6.409) (218.0301, 5.7663) knots 0 0 0 0 1 1 1 1
  spline S1066 degree 3 poles (218.0301, 5.7663) (218.0346, 5.6813) (217.9334, 5.6209) (217.9172, 5.5373) knots 0 0 0 0 1 1 1 1
  spline S1067 degree 3 poles (217.9172, 5.5373) (217.8752, 5.3208) (217.8697, 5.0986) (217.8579, 4.8784) knots 0 0 0 0 1 1 1 1
  spline S1068 degree 3 poles (217.8579, 4.8784) (217.8354, 4.4618) (217.7994, 4.0446) (217.8144, 3.6277) knots 0 0 0 0 1 1 1 1
  spline S1069 degree 3 poles (217.8144, 3.6277) (217.8218, 3.4219) (217.9208, 3.2258) (217.9248, 3.02) knots 0 0 0 0 1 1 1 1
  spline S1070 degree 3 poles (217.9248, 3.02) (217.9296, 2.776) (217.804, 2.534) (217.8405, 2.2926) knots 0 0 0 0 1 1 1 1
  spline S1071 degree 3 poles (217.8405, 2.2926) (217.9551, 1.5341) (218.1955, 0.7999) (218.3731, 0.0536) knots 0 0 0 0 1 1 1 1
  spline S1072 degree 3 poles (217.8948, 9.6429) (217.6601, 10.1381) (217.3333, 10.5994) (217.1906, 11.1285) knots 0 0 0 0 1 1 1 1
  spline S1073 degree 3 poles (217.1906, 11.1285) (216.5322, 13.57) (216.0986, 16.0669) (215.4998, 18.5237) knots 0 0 0 0 1 1 1 1
  spline S1074 degree 3 poles (215.4998, 18.5237) (215.4274, 18.8205) (215.2492, 19.0848) (215.179, 19.3821) knots 0 0 0 0 1 1 1 1
  spline S1075 degree 3 poles (215.179, 19.3821) (214.9076, 20.5316) (214.783, 21.7144) (214.477, 22.8552) knots 0 0 0 0 1 1 1 1
  spline S1076 degree 3 poles (214.477, 22.8552) (214.1697, 24.0005) (213.7208, 25.1029) (213.3426, 26.2267) knots 0 0 0 0 1 1 1 1
  spline S1077 degree 3 poles (213.3073, 29.48) (213.3043, 27.8658) (213.0229, 26.228) (213.2984, 24.6375) knots 0 0 0 0 1 1 1 1
  spline S1078 degree 3 poles (213.2984, 24.6375) (214.1557, 19.6888) (215.2556, 14.7702) (216.6893, 9.9568) knots 0 0 0 0 1 1 1 1
  spline S1079 degree 3 poles (216.6893, 9.9568) (216.9217, 9.1764) (217.7518, 8.7206) (218.2345, 8.0648) knots 0 0 0 0 1 1 1 1
  spline S1080 degree 3 poles (218.2345, 8.0648) (218.3494, 7.9086) (218.4211, 7.7209) (218.4724, 7.5339) knots 0 0 0 0 1 1 1 1
  spline S1081 degree 3 poles (218.4724, 7.5339) (218.5544, 7.2352) (218.6013, 6.9267) (218.6313, 6.6184) knots 0 0 0 0 1 1 1 1
  spline S1082 degree 3 poles (218.6313, 6.6184) (218.719, 5.7169) (218.7239, 4.8081) (218.8252, 3.908) knots 0 0 0 0 1 1 1 1
  spline S1083 degree 3 poles (218.8252, 3.908) (218.8416, 3.7625) (218.9004, 3.6191) (218.9824, 3.4977) knots 0 0 0 0 1 1 1 1
  spline S1084 degree 3 poles (218.9824, 3.4977) (219.0731, 3.3634) (219.215, 3.2718) (219.3313, 3.1588) knots 0 0 0 0 1 1 1 1
  spline S1085 degree 3 poles (213.1219, 31.6607) (213.1219, 31.7585) (213.1219, 31.8562) (213.1219, 31.954) knots 0 0 0 0 1 1 1 1
  spline S1086 degree 3 poles (213.7788, 30.4932) (213.7084, 30.8423) (213.6625, 31.1972) (213.5677, 31.5405) knots 0 0 0 0 1 1 1 1
  spline S1087 degree 3 poles (213.5677, 31.5405) (213.5273, 31.6869) (213.5139, 31.8907) (213.3756, 31.9536) knots 0 0 0 0 1 1 1 1
  spline S1088 degree 3 poles (213.3756, 31.9536) (213.1554, 32.0537) (212.8917, 31.9564) (212.6498, 31.9578) knots 0 0 0 0 1 1 1 1
  spline S1089 degree 3 poles (213.188, 41.3576) (212.9933, 41.3803) (212.7994, 41.4409) (212.604, 41.4257) knots 0 0 0 0 1 1 1 1
  spline S1090 degree 3 poles (212.604, 41.4257) (212.5324, 41.4202) (212.4438, 41.3694) (212.4297, 41.299) knots 0 0 0 0 1 1 1 1
  spline S1091 degree 3 poles (212.4297, 41.299) (212.3735, 41.0173) (212.3997, 40.7247) (212.4069, 40.4375) knots 0 0 0 0 1 1 1 1
  spline S1092 degree 3 poles (212.4069, 40.4375) (212.5181, 36.0326) (212.6459, 31.6282) (212.7848, 27.2241) knots 0 0 0 0 1 1 1 1
  spline S1093 degree 3 poles (212.7848, 27.2241) (212.795, 26.8998) (212.7911, 26.5715) (212.8543, 26.2532) knots 0 0 0 0 1 1 1 1
  spline S1094 degree 3 poles (212.8543, 26.2532) (212.9631, 25.7054) (213.1504, 25.1761) (213.2984, 24.6375) knots 0 0 0 0 1 1 1 1
  spline S1095 degree 3 poles (222.8286, 154.7911) (222.6654, 154.5546) (222.5022, 154.3182) (222.339, 154.0818) knots 0 0 0 0 1 1 1 1
  spline S1096 degree 3 poles (225.8139, 27.7151) (225.6275, 27.7471) (225.4203, 27.7197) (225.2548, 27.8111) knots 0 0 0 0 1 1 1 1
  spline S1097 degree 3 poles (225.2548, 27.8111) (225.0436, 27.9277) (224.9068, 28.1452) (224.7329, 28.3123) knots 0 0 0 0 1 1 1 1
  spline S1098 degree 3 poles (59.8508, 32.5406) (59.8505, 31.7787) (59.8502, 31.0167) (59.8499, 30.2548) knots 0 0 0 0 1 1 1 1
  spline S1099 degree 3 poles (59.716, 69.8143) (59.716, 70.9846) (59.716, 72.155) (59.716, 73.3253) knots 0 0 0 0 1 1 1 1